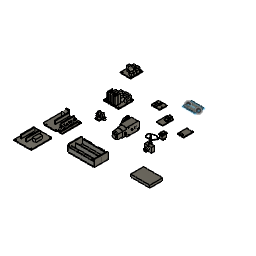
RoboCar2Lib (Autodesk Fusion 360 design; units mm, degrees)
Autodesk Fusion 360 part; units mm, degrees
(part 1 of 2)
sketch "Sketch1" plane through (0, 0, 0) normal (0, 1, 0) x (1, 0, 0)
  line L0 (25, -36.5) -> (33.5, -36.5)
  line L1 (33.5, -36.5) -> (33.5, -13.5)
  line L2 (33.5, -13.5) -> (25, -13.5)
  line L3 (25.0032, -15) -> (25, -15)
  line L4 (32.5, -31.6144) -> (32.5, -18.3856)
  line L5 (25, -36.5) -> (14.5, -36.5)
  line L6 (14.5, -36.5) -> (14.5, -13.5)
  line L7 (14.5, -13.5) -> (25, -13.5)
  line L8 (25, -36.5) -> (16.5, -36.5)
  line L9 (16.5, -32.746) -> (16.5, -17.254)
  line L10 (16.5, -13.5) -> (25, -13.5)
  arc A0 (32.5, -18.3856) -> (17.5, -18.3856) centre (25, -25) ccw
  arc A1 (17.5, -31.6144) -> (32.5, -31.6144) centre (25, -25) ccw
  arc A2 (33.5, -17.254) -> (16.5, -17.254) centre (25, -25) ccw
  arc A3 (16.5, -32.746) -> (33.5, -32.746) centre (25, -25) ccw
  line L11 (17.5, -31.6144) -> (17.5, -18.3856)
  circle A4 centre (25, -25) radius 5
  dimension "d1" = 20
  dimension "d2" = 23
  dimension "d3" = 8.5
  dimension "d4" = 23
  dimension "d7" = 10.5
  dimension "d8" = 23
  dimension "d16" = 10
  constraint concentric A0 A2
  constraint horizontal L0
  constraint vertical L1
  constraint horizontal L2
  constraint coincident L0.start A2
  constraint horizontal L3
  constraint coincident L1 A3.end
  constraint coincident L1 A2.start
  constraint coincident L3.start A0
  constraint horizontal L5
  constraint vertical L6
  constraint horizontal L7
  constraint horizontal L8
  constraint vertical L9
  constraint horizontal L10
  constraint concentric A0 A1
  constraint concentric A2 A3
  constraint concentric A3 A4
  measures "d1" diameter of A0
  measures "d2" diameter of A2
  measures "d3" distance of L0.start L0.end
  measures "d4" distance of L0.start L2.end
  measures "d7" distance of L0.start L5.end
  measures "d8" distance of L0.start L2.end
  measures "d16" diameter of A4
extrude "Extrude1" add sketch "Sketch1" against normal blind 25 contours L3 L4 A0 A1 L11 | A4 makes body 1
extrude "Extrude2" add sketch "Sketch1" against normal blind 11 contours L1 L9 A2 A3 bodies 1
extrude "Extrude3" add sketch "Sketch1" along normal blind 37 contours L0 L1 A3 | L5 L6 L7 L8 L9 L10 A2 A3 | L1 L9 A2 A3 | L1 L2 A2 | L3 L4 A0 A1 L11 | A4 bodies 1
extrude "Extrude4" add sketch "Sketch1" against normal blind 28 contours A4 bodies 1
fillet "Fillet1" radius 4 1 edges at (24, 37, 36.5) on bodies 1
fillet "Fillet2" radius 4 1 edges at (24, 37, 13.5) on bodies 1
sketch "Sketch2" plane through (33.5, 0, 0) normal (1, 0, 0) x (0, 1, 0)
  arc A0 (33, 13.5) -> (37, 17.5) centre (33, 17.5) ccw
  line L0 (37, 17.5) -> (37, 32.5)
  arc A1 (37, 32.5) -> (33, 36.5) centre (33, 32.5) ccw
  line L1 (33, 36.5) -> (0, 36.5)
  line L2 (0, 36.5) -> (0, 32.746)
  line L3 (0, 32.746) -> (-11, 32.746)
  line L4 (-11, 32.746) -> (-11, 17.254)
  line L5 (-11, 17.254) -> (0, 17.254)
  line L6 (0, 17.254) -> (0, 13.5)
  line L7 (0, 13.5) -> (33, 13.5)
  line L8 (0, 36.5) -> (0, 13.5)
  circle A2 centre (14.5, 25) radius 2
  line L9 (0, 25) -> (25.5, 25)
  circle A3 centre (25.5, 25) radius 2.75
  line L10 (0, 25) -> (-11, 25)
  line L11 (-6.5, 27.5) -> (-3.5, 27.5)
  line L12 (-3.5, 27.5) -> (-3.5, 22.5)
  line L13 (-3.5, 22.5) -> (-6.5, 22.5)
  line L14 (-6.5, 22.5) -> (-6.5, 27.5)
  circle A4 centre (5.5, 34) radius 1.5
  circle A5 centre (5.5, 16) radius 1.5
  dimension "d23" = 4
  dimension "d24" = 25.5
  dimension "d25" = 5.5
  dimension "d32" = 4.5
  dimension "d33" = 3
  dimension "d34" = 2.5
  dimension "d35" = 2.5
  dimension "d44" = 3
  dimension "d45" = 5.5
  dimension "d46" = 2.5
  dimension "d47" = 3
  dimension "d48" = 5.5
  dimension "d49" = 2.5
  constraint midpoint L8 L9.start
  constraint perpendicular L8 L9
  constraint coincident L9.end A3.centre
  constraint midpoint L4 L10.end
  constraint horizontal L11
  constraint vertical L12
  constraint horizontal L13
  constraint vertical L14
  measures "d23" diameter of A2
  measures "d24" distance of L9.start L9.end
  measures "d25" diameter of A3
  measures "d32" distance of L4 L14
  measures "d33" distance of L12 L14
  measures "d34" distance of L10 L11
  measures "d35" distance of L10 L13
  measures "d44" diameter of A4
  measures "d45" distance of L8 A4.centre
  measures "d46" distance of L1 A4.centre
  measures "d47" diameter of A5
  measures "d48" distance of L8 A5.centre
  measures "d49" distance of L7 A5.centre
extrude "Extrude5" add sketch "Sketch2" along normal blind 2 contours A2 L9 | A2 L9 bodies 1
extrude "Extrude6" add sketch "Sketch2" along normal blind 8 contours A3 bodies 1
extrude "Extrude7" add sketch "Sketch2" against normal blind 28 contours A3 bodies 1
extrude "Extrude8" add sketch "Sketch2" along normal blind 2.5 contours L10 L12 L13 L14 | L10 L11 L12 L14 bodies 1
extrude "Extrude9" add sketch "Sketch2" against normal blind 19.5 contours L10 L12 L13 L14 | L10 L11 L12 L14 bodies 1
fillet "Fillet3" radius 2 1 edges at (25, -25, 35) on bodies 1
fillet "Fillet4" radius 2 1 edges at (25, -25, 15) on bodies 1
copy_body "Body->Comp1" bodies 1 removing the originals makes body 2 in component "MotorReductor"
extrude "Extrude1'" cut sketch "Sketch2" against normal blind 39 contours A4 | A5 bodies 2 in component "MotorReductor"
sketch "Sketch3" plane through (0, 37, 0) normal (0, 1, 0) x (-1, 0, 0)
  line L0 (-33.5, 17.5) -> (-14.5, 17.5)
  line L1 (-14.5, 17.5) -> (-14.5, 32.5)
  line L2 (-14.5, 32.5) -> (-33.5, 32.5)
  line L3 (-33.5, 32.5) -> (-33.5, 17.5)
  line L4 (-26.5, 27.5) -> (-23.5, 27.5)
  line L5 (-23.5, 27.5) -> (-23.5, 22.5)
  line L6 (-23.5, 22.5) -> (-26.5, 22.5)
  line L7 (-26.5, 22.5) -> (-26.5, 27.5)
  point P0 (-25, 25)
  dimension "d52" = 1.5
  dimension "d53" = 1.5
  dimension "d54" = 2.5
  dimension "d55" = 2.5
  constraint horizontal L4
  constraint vertical L5
  constraint horizontal L6
  constraint vertical L7
  measures "d52" distance of P0 L7
  measures "d53" distance of P0 L5
  measures "d54" distance of P0 L4
  measures "d55" distance of P0 L6
extrude "Extrude2'" add sketch "Sketch3" along normal blind 5 contours L4 L5 L6 L7 bodies 2 in component "MotorReductor"
sketch "Sketch4" plane through (26.5, 0, 0) normal (1, 0, 0) x (0, 1, 0)
  line L0 (37, 27.5) -> (37, 22.5)
  line L1 (37, 22.5) -> (42, 22.5)
  line L2 (42, 22.5) -> (42, 27.5)
  line L3 (42, 27.5) -> (37, 27.5)
  circle A0 centre (39.5, 25) radius 1.5
  dimension "d58" = 3
  measures "d58" diameter of A0
extrude "Extrude3'" cut sketch "Sketch4" against normal blind 9.5 contours A0 bodies 2 in component "MotorReductor"
sketch "Sketch5" plane through (5.5, 0, 0) normal (-1, 0, 0) x (0, -1, 0)
  circle A0 centre (-25.5, 25) radius 2.75
  circle A1 centre (-25.5, 25) radius 13
  line L0 (-26, 36) -> (-25, 36)
  line L1 (-25, 36) -> (-25, 32)
  line L2 (-25, 32) -> (-26, 32)
  line L3 (-26, 32) -> (-26, 36)
  line L4 (-28.1386, 31.5029) -> (-29.3747, 35.3071)
  line L5 (-28.4237, 35.6161) -> (-27.1876, 31.8119)
  line L6 (-29.3747, 35.3071) -> (-28.4237, 35.6161)
  line L7 (-27.1876, 31.8119) -> (-28.1386, 31.5029)
  line L8 (-30.019, 30.3692) -> (-32.3701, 33.6053)
  line L9 (-31.5611, 34.1931) -> (-29.21, 30.957)
  line L10 (-32.3701, 33.6053) -> (-31.5611, 34.1931)
  line L11 (-29.21, 30.957) -> (-30.019, 30.3692)
  line L12 (-31.457, 28.71) -> (-34.6931, 31.0611)
  line L13 (-34.1053, 31.8701) -> (-30.8692, 29.519)
  line L14 (-34.6931, 31.0611) -> (-34.1053, 31.8701)
  line L15 (-30.8692, 29.519) -> (-31.457, 28.71)
  line L16 (-32.3119, 26.6876) -> (-36.1161, 27.9237)
  line L17 (-35.8071, 28.8747) -> (-32.0029, 27.6386)
  line L18 (-36.1161, 27.9237) -> (-35.8071, 28.8747)
  line L19 (-32.0029, 27.6386) -> (-32.3119, 26.6876)
  line L20 (-32.5, 24.5) -> (-36.5, 24.5)
  line L21 (-36.5, 25.5) -> (-32.5, 25.5)
  line L22 (-36.5, 24.5) -> (-36.5, 25.5)
  line L23 (-32.5, 25.5) -> (-32.5, 24.5)
  line L24 (-32.0029, 22.3614) -> (-35.8071, 21.1253)
  line L25 (-36.1161, 22.0763) -> (-32.3119, 23.3124)
  line L26 (-35.8071, 21.1253) -> (-36.1161, 22.0763)
  line L27 (-32.3119, 23.3124) -> (-32.0029, 22.3614)
  line L28 (-30.8692, 20.481) -> (-34.1053, 18.1299)
  line L29 (-34.6931, 18.9389) -> (-31.457, 21.29)
  line L30 (-34.1053, 18.1299) -> (-34.6931, 18.9389)
  line L31 (-31.457, 21.29) -> (-30.8692, 20.481)
  line L32 (-29.21, 19.043) -> (-31.5611, 15.8069)
  line L33 (-32.3701, 16.3947) -> (-30.019, 19.6308)
  line L34 (-31.5611, 15.8069) -> (-32.3701, 16.3947)
  line L35 (-30.019, 19.6308) -> (-29.21, 19.043)
  line L36 (-27.1876, 18.1881) -> (-28.4237, 14.3839)
  line L37 (-29.3747, 14.6929) -> (-28.1386, 18.4971)
  line L38 (-28.4237, 14.3839) -> (-29.3747, 14.6929)
  line L39 (-28.1386, 18.4971) -> (-27.1876, 18.1881)
  line L40 (-25, 18) -> (-25, 14)
  line L41 (-26, 14) -> (-26, 18)
  line L42 (-25, 14) -> (-26, 14)
  line L43 (-26, 18) -> (-25, 18)
  line L44 (-22.8614, 18.4971) -> (-21.6253, 14.6929)
  line L45 (-22.5763, 14.3839) -> (-23.8124, 18.1881)
  line L46 (-21.6253, 14.6929) -> (-22.5763, 14.3839)
  line L47 (-23.8124, 18.1881) -> (-22.8614, 18.4971)
  line L48 (-20.981, 19.6308) -> (-18.6299, 16.3947)
  line L49 (-19.4389, 15.8069) -> (-21.79, 19.043)
  line L50 (-18.6299, 16.3947) -> (-19.4389, 15.8069)
  line L51 (-21.79, 19.043) -> (-20.981, 19.6308)
  line L52 (-19.543, 21.29) -> (-16.3069, 18.9389)
  line L53 (-16.8947, 18.1299) -> (-20.1308, 20.481)
  line L54 (-16.3069, 18.9389) -> (-16.8947, 18.1299)
  line L55 (-20.1308, 20.481) -> (-19.543, 21.29)
  line L56 (-18.6881, 23.3124) -> (-14.8839, 22.0763)
  line L57 (-15.1929, 21.1253) -> (-18.9971, 22.3614)
  line L58 (-14.8839, 22.0763) -> (-15.1929, 21.1253)
  line L59 (-18.9971, 22.3614) -> (-18.6881, 23.3124)
  line L60 (-18.5, 25.5) -> (-14.5, 25.5)
  line L61 (-14.5, 24.5) -> (-18.5, 24.5)
  line L62 (-14.5, 25.5) -> (-14.5, 24.5)
  line L63 (-18.5, 24.5) -> (-18.5, 25.5)
  line L64 (-18.9971, 27.6386) -> (-15.1929, 28.8747)
  line L65 (-14.8839, 27.9237) -> (-18.6881, 26.6876)
  line L66 (-15.1929, 28.8747) -> (-14.8839, 27.9237)
  line L67 (-18.6881, 26.6876) -> (-18.9971, 27.6386)
  line L68 (-20.1308, 29.519) -> (-16.8947, 31.8701)
  line L69 (-16.3069, 31.0611) -> (-19.543, 28.71)
  line L70 (-16.8947, 31.8701) -> (-16.3069, 31.0611)
  line L71 (-19.543, 28.71) -> (-20.1308, 29.519)
  line L72 (-21.79, 30.957) -> (-19.4389, 34.1931)
  line L73 (-18.6299, 33.6053) -> (-20.981, 30.3692)
  line L74 (-19.4389, 34.1931) -> (-18.6299, 33.6053)
  line L75 (-20.981, 30.3692) -> (-21.79, 30.957)
  line L76 (-23.8124, 31.8119) -> (-22.5763, 35.6161)
  line L77 (-21.6253, 35.3071) -> (-22.8614, 31.5029)
  line L78 (-22.5763, 35.6161) -> (-21.6253, 35.3071)
  line L79 (-22.8614, 31.5029) -> (-23.8124, 31.8119)
  dimension "d61" = 26
  dimension "d65" = 360
  constraint concentric A0 A1
  constraint horizontal L0
  constraint vertical L1
  constraint horizontal L2
  constraint vertical L3
  measures "d61" diameter of A1
extrude "Extrude4'" add sketch "Sketch5" against normal blind 3 contours A1 | L0 L1 L2 L3 | L4 L5 L6 L7 | L8 L9 L10 L11 | L12 L13 L14 L15 | L16 L17 L18 L19 | L20 L21 L22 L23 | L24 L25 L26 L27 | L28 L29 L30 L31 | L32 L33 L34 L35 | L36 L37 L38 L39 | L40 L41 L42 L43 | L44 L45 L46 L47 | L48 L49 L50 L51 | L52 L53 L54 L55 | L56 L57 L58 L59 | L60 L61 L62 L63 | L64 L65 L66 L67 | L68 L69 L70 L71 | L72 L73 L74 L75 | L76 L77 L78 L79 bodies 2 in component "MotorReductor"
delete_face "DeleteFace1" 1 faces at (8.5, 15.9753, 24.2175) on bodies 2 in component "MotorReductor"
extrude "Extrude5'" add sketch "Sketch5" against normal blind 3 bodies 2 in component "MotorReductor"
sketch "Sketch6" plane through (0, 0, 0) normal (0, 0, 1) x (1, 0, 0)
  circle A0 centre (-75, 25) radius 1.5
  line L0 (-65, 40) -> (-65, 9)
  line L1 (-75, 21.75) -> (-71, 21.75)
  line L2 (-65, 21.75) -> (-65, 28.25)
  line L3 (-65, 28.25) -> (-75, 28.25)
  line L4 (-65, 21.75) -> (-71, 21.75)
  line L5 (-71, 21.75) -> (-71, 13.75)
  line L6 (-71, 13.75) -> (-65, 13.75)
  line L7 (-65, 13.75) -> (-65, 21.75)
  line L8 (-68, 28.25) -> (-68, 21.75)
  line L9 (-72, 28.25) -> (-72, 21.75)
  arc A1 (-75, 28.25) -> (-75, 21.75) centre (-75, 25) ccw
  circle A2 centre (-69.4791, 26.484) radius 0.8565
  circle A3 centre (-69.4791, 23.583) radius 0.8405
  line L10 (-68.6088, 20.0696) -> (-70.0915, 20.0696)
  line L11 (-70.0915, 20.0696) -> (-70.0915, 17.5876)
  line L12 (-70.0915, 17.5876) -> (-68.6088, 17.5876)
  line L13 (-68.6088, 17.5876) -> (-68.6088, 20.0696)
  line L14 (-66, 16) -> (-70.0593, 16)
  line L15 (-70.0593, 16) -> (-70.0593, 14.6866)
  line L16 (-70.0593, 14.6866) -> (-66, 14.6866)
  line L17 (-66, 14.6866) -> (-66, 16)
  dimension "d68" = 3
  dimension "d69" = 10
  dimension "d70" = 6.5
  dimension "d71" = 6.5
  dimension "d72" = 6
  dimension "d73" = 8
  dimension "d74" = 3
  dimension "d75" = 4
  constraint vertical L0
  constraint concentric A0 A1
  constraint horizontal L1
  constraint vertical L2
  constraint horizontal L3
  constraint horizontal L4
  constraint vertical L5
  constraint horizontal L6
  constraint vertical L7
  constraint coincident L3 L8.start
  constraint coincident L4 L8.end
  constraint perpendicular L4 L8
  constraint coincident L3 L9.start
  constraint coincident L1 L9.end
  constraint perpendicular L1 L9
  constraint horizontal L10
  constraint vertical L11
  constraint horizontal L12
  constraint vertical L13
  constraint horizontal L14
  constraint vertical L15
  constraint horizontal L16
  constraint vertical L17
  measures "d68" diameter of A0
  measures "d69" distance of A0.centre L0
  measures "d70" diameter of A1
  measures "d71" distance of L1.start L3.end
  measures "d72" distance of L2.start L1.end
  measures "d73" distance of L2.start L6.end
  measures "d74" distance of L0 L8
  measures "d75" distance of L8 L9
extrude "Extrude10" add sketch "Sketch6" along normal blind 4.5 separate body contours L1 L3 L9 A1 makes body 3
extrude "Extrude11" add sketch "Sketch6" along normal blind 5 separate body contours L0 L2 L3 L4 L8 makes body 4
extrude "Extrude12" add sketch "Sketch6" along normal blind 13 contours L1 L3 L4 L8 L9 | A2 | A3 bodies 3 4
extrude "Extrude13" add sketch "Sketch6" along normal blind 1.6 contours L0 L4 L5 L6 L7 | L10 L11 L12 L13 | L14 L15 L16 L17 bodies 3
extrude "Extrude14" add sketch "Sketch6" against normal blind 1.3 contours A2 | A3 | L10 L11 L12 L13 | L14 L15 L16 L17 bodies 3
mirror "Mirror1" about plane through (-65, 21.75, 0) normal (1, 0, 0) of bodies 3 merged
copy_body "Body->Comp2" bodies 3 removing the originals makes body 5 in component "Encoder"
sketch "Sketch7" plane through (0, 0, 0) normal (0, 0, 1) x (1, 0, 0)
  line L0 (-26.5653, -67.5474) -> (49.4347, -67.5474)
  line L1 (49.4347, -67.5474) -> (49.4347, -108.5474)
  line L2 (49.4347, -108.5474) -> (-26.5653, -108.5474)
  line L3 (-26.5653, -108.5474) -> (-26.5653, -67.5474)
  line L4 (47.4347, -67.5474) -> (47.4347, -108.5474)
  line L5 (-24.5653, -67.5474) -> (-24.5653, -108.5474)
  dimension "d88" = 76
  dimension "d89" = 41
  dimension "d90" = 2
  dimension "d91" = 2
  constraint horizontal L0
  constraint vertical L1
  constraint horizontal L2
  constraint vertical L3
  constraint perpendicular L2 L4
  constraint coincident L0 L4.start
  constraint coincident L2 L4.end
  constraint vertical L5
  constraint coincident L0 L5.start
  constraint coincident L2 L5.end
  measures "d88" distance of L0.start L0.end
  measures "d89" distance of L0.start L2.end
  measures "d90" distance of L1 L4
  measures "d91" distance of L3 L5
extrude "Extrude15" add sketch "Sketch7" along normal blind 20 separate body contours L0 L2 L3 L5 | L0 L1 L2 L4 makes body 6 at (-24.5653, -81.2141, 6.6667) makes body 7 at (49.4347, -81.2141, 6.6667)
extrude "Extrude16" add sketch "Sketch7" along normal blind 2 contours L0 L2 L4 L5 bodies 6 7
fillet "Fillet5" radius 4 4 edges at (48.4347, -108.5474, 20) (-25.5653, -108.5474, 20) (48.4347, -67.5474, 20) (-25.5653, -67.5474, 20) on bodies 6
sketch "Sketch8" plane through (-26.5653, 0, 0) normal (-1, 0, 0) x (0, -1, 0)
  arc A0 (71.5474, 20) -> (67.5474, 16) centre (71.5474, 16) ccw
  line L0 (67.5474, 16) -> (67.5474, 0)
  line L1 (67.5474, 0) -> (108.5474, 0)
  line L2 (108.5474, 0) -> (108.5474, 16)
  arc A1 (108.5474, 16) -> (104.5474, 20) centre (104.5474, 16) ccw
  line L3 (104.5474, 20) -> (71.5474, 20)
  line L4 (108.5474, 0) -> (107.0474, 0)
  line L5 (107.0474, 0) -> (107.0474, 14)
  line L6 (108.5474, 14) -> (108.5474, 0)
  line L7 (67.5474, 0) -> (69.0474, 0)
  line L8 (69.0474, 0) -> (69.0474, 14)
  line L9 (67.5474, 14) -> (67.5474, 0)
  arc A2 (70.1082, 18.3088) -> (67.5474, 14) centre (72.4529, 14) ccw
  arc A3 (70.7763, 16.9642) -> (69.0474, 14) centre (72.4529, 14) ccw
  line L10 (70.6663, 18.1167) -> (70.9463, 17.4716)
  arc A4 (70.6663, 18.1167) -> (70.1082, 18.3088) centre (70.2994, 17.9575) ccw
  arc A5 (70.7763, 16.9642) -> (70.9463, 17.4716) centre (70.5794, 17.3123) ccw
  line L11 (88.0474, 20) -> (88.0474, 0)
  arc A6 (108.5474, 14) -> (105.9866, 18.3088) centre (103.6419, 14) ccw
  arc A7 (107.0474, 14) -> (105.3185, 16.9642) centre (103.6419, 14) ccw
  arc A8 (105.9866, 18.3088) -> (105.4285, 18.1167) centre (105.7955, 17.9575) ccw
  line L12 (105.4285, 18.1167) -> (105.1485, 17.4716)
  arc A9 (105.1485, 17.4716) -> (105.3185, 16.9642) centre (105.5155, 17.3123) ccw
  line L13 (87.3474, 14) -> (88.7474, 14)
  line L14 (108.5474, 0) -> (67.5474, 0)
  line L15 (88.7474, 14) -> (88.7474, 0)
  line L16 (87.3474, 14) -> (87.3474, 0)
  dimension "d98" = 1.5
  dimension "d99" = 14
  dimension "d100" = 1.5
  dimension "d102" = 0.4
  dimension "d103" = 20.5
  dimension "d106" = 14
  constraint horizontal L4
  constraint vertical L5
  constraint vertical L6
  constraint coincident L1.end L2.start
  constraint horizontal L7
  constraint vertical L8
  constraint vertical L9
  constraint coincident L0.end L1.start
  constraint tangent L9 A2
  constraint concentric A2 A3
  constraint tangent A2 A4
  constraint tangent L10 A4
  constraint tangent A3 A5
  constraint tangent L10 A5
  constraint equal A4 A5
  constraint perpendicular L1 L11
  constraint symmetric L9.start L11 L6.start
  constraint symmetric A2 L11 A6
  constraint symmetric L8.end L11 L5.end
  constraint symmetric A3 L11 A7
  constraint symmetric L10.start L11 A8.end
  constraint symmetric A2.start L11 A6.end
  constraint symmetric A4 L11 A8
  constraint symmetric L10.end L11 L12.end
  constraint symmetric A3.start L11 A7.end
  constraint symmetric A5 L11 A9
  constraint coincident L1 L11.end
  constraint coincident L3 L11.start
  constraint coincident L1 L15.end
  constraint coincident L1 L16.end
  measures "d98" distance of L1.end L4.end
  measures "d99" distance of L1.end L6.start
  measures "d100" distance of L0.end L7.end
  measures "d102" radius of A4
  measures "d103" distance of L9 L11
  measures "d106" distance of L13 L14
extrude "Extrude17" add sketch "Sketch8" against normal blind 74 contours L0 L1 L7 L8 L9 A2 A3 L10 A4 A5 L14 | L1 L11 L13 L14 L15 | L1 L11 L13 L14 L16 | L1 L2 L4 L5 L6 A6 A7 A8 L12 A9 L14 bodies 6
sketch "Sketch9" plane through (0, -108.5474, 0) normal (0, -1, 0) x (1, 0, 0)
  line L0 (-24.5653, 14) -> (-24.5653, 16)
  line L1 (-24.5653, 16) -> (-26.5653, 16)
  line L2 (-26.5653, 16) -> (-26.5653, 0)
  line L3 (-26.5653, 0) -> (49.4347, 0)
  line L4 (49.4347, 0) -> (49.4347, 16)
  line L5 (49.4347, 16) -> (47.4347, 16)
  line L6 (47.4347, 16) -> (47.4347, 14)
  line L7 (47.4347, 14) -> (-24.5653, 14)
  line L8 (4.284, 14) -> (18.5854, 14)
  line L9 (49.4347, 0) -> (-26.5653, 0)
  line L10 (3.4347, 14.2636) -> (3.4347, 14)
  line L11 (19.4347, 14.2636) -> (19.4347, 14)
  line L12 (0.4347, 19) -> (2.9978, 14.7283)
  line L13 (22.4347, 19) -> (19.8717, 14.7283)
  arc A0 (2.9978, 14.7283) -> (4.284, 14) centre (4.284, 15.5) ccw
  arc A1 (18.5854, 14) -> (19.8717, 14.7283) centre (18.5854, 15.5) ccw
  line L14 (0.4347, 19) -> (22.4347, 19)
  line L15 (-26.5653, 16) -> (-26.5653, 20)
  line L16 (-18.5653, 17) -> (-18.5653, 20)
  line L17 (-18.5653, 20) -> (-24.5653, 20)
  line L18 (-24.5653, 20) -> (-24.5653, 17)
  arc A2 (-24.5653, 17) -> (-18.5653, 17) centre (-21.5653, 17) ccw
  line L19 (47.4347, 17) -> (47.4347, 20)
  line L20 (47.4347, 20) -> (41.4347, 20)
  line L21 (41.4347, 20) -> (41.4347, 17)
  arc A3 (41.4347, 17) -> (47.4347, 17) centre (44.4347, 17) ccw
  dimension "d109" = 14
  dimension "d115" = 1.5
  dimension "d116" = 6
  dimension "d117" = 5
  dimension "d118" = 6
  dimension "d119" = 6
  dimension "d120" = 5
  dimension "d121" = 6
  dimension "d122" = 3
  constraint horizontal L8
  constraint vertical L10
  constraint vertical L11
  constraint tangent L12 A0
  constraint tangent L8 A0
  constraint tangent L13 A1
  constraint tangent L8 A1
  constraint equal A0 A1
  constraint coincident A0 L10.start
  constraint coincident L7 L10.end
  constraint coincident L7 L11.end
  constraint coincident A1 L11.start
  constraint vertical L16
  constraint horizontal L17
  constraint vertical L18
  constraint vertical L19
  constraint horizontal L20
  constraint vertical L21
  measures "d109" distance of L8 L9
  measures "d115" radius of A0
  measures "d116" diameter of A2
  measures "d117" distance of A2.centre L15
  measures "d118" distance of L18.end L16.start
  measures "d119" diameter of A3
  measures "d120" distance of L4 A3.centre
  measures "d121" distance of L21.end L19.start
  measures "d122" distance of L21.end L20.end
extrude "Extrude18" cut sketch "Sketch9" against normal blind 45 contours L16 L17 L18 A2 | L19 L20 L21 A3 | L7 L8 L12 L13 A0 A1 L14 bodies 6
copy_body "Body->Comp3" bodies 6 removing the originals makes body 8 in component "BattaryHolder"
sketch "Sketch10" plane through (0, 0, 0) normal (0, 0, 1) x (1, 0, 0)
  line L0 (-134.5632, -15) -> (-80.9632, -15)
  line L1 (-80.9632, -15) -> (-80.9632, -70)
  line L2 (-97.4, -73) -> (-130, -73)
  line L3 (-134.5632, -70) -> (-134.5632, -15)
  line L4 (-130, -73) -> (-133, -70)
  line L5 (-94.4, -70) -> (-97.4, -73)
  line L6 (-94.4, -70) -> (-98.6426, -70) construction
  line L7 (-134.5632, -70) -> (-133, -70)
  line L8 (-94.4, -70) -> (-80.9632, -70)
  circle A0 centre (-131.5632, -19.5) radius 1.5
  circle A1 centre (-83.9632, -19.5) radius 1.5
  circle A2 centre (-126.5632, -70.5) radius 1.5
  circle A3 centre (-98.9632, -70.5) radius 1.5
  line L9 (-127.5632, -12) -> (-118.5632, -12)
  line L10 (-118.5632, -12) -> (-118.5632, -26)
  line L11 (-118.5632, -26) -> (-127.5632, -26)
  line L12 (-127.5632, -26) -> (-127.5632, -12)
  line L13 (-116.0632, -17.5) -> (-113.5632, -17.5)
  line L14 (-113.5632, -17.5) -> (-113.5632, -56.5)
  line L15 (-113.5632, -56.5) -> (-116.0632, -56.5)
  line L16 (-116.0632, -56.5) -> (-116.0632, -17.5)
  line L17 (-100.5632, -17.5) -> (-98.0632, -17.5)
  line L18 (-98.0632, -17.5) -> (-98.0632, -56.5)
  line L19 (-98.0632, -56.5) -> (-100.5632, -56.5)
  line L20 (-100.5632, -56.5) -> (-100.5632, -17.5)
  line L21 (-93.9632, -20) -> (-86.4632, -20)
  line L22 (-86.4632, -20) -> (-86.4632, -30)
  line L23 (-86.4632, -30) -> (-93.9632, -30)
  line L24 (-93.9632, -30) -> (-93.9632, -20)
  circle A4 centre (-92.7132, -21.25) radius 0.5
  circle A5 centre (-90.2132, -21.25) radius 0.5
  circle A6 centre (-87.7132, -21.25) radius 0.5
  circle A7 centre (-92.7132, -23.75) radius 0.5
  circle A8 centre (-90.2132, -23.75) radius 0.5
  circle A9 centre (-87.7132, -23.75) radius 0.5
  circle A10 centre (-92.7132, -26.25) radius 0.5
  circle A11 centre (-90.2132, -26.25) radius 0.5
  circle A12 centre (-87.7132, -26.25) radius 0.5
  circle A13 centre (-92.7132, -28.75) radius 0.5
  circle A14 centre (-90.2132, -28.75) radius 0.5
  circle A15 centre (-87.7132, -28.75) radius 0.5
  dimension "d125" = 53.6
  dimension "d126" = 58
  dimension "d127" = 3
  dimension "d129" = 45
  dimension "d130" = 3
  dimension "d131" = 3
  dimension "d132" = 3
  dimension "d133" = 3
  dimension "d134" = 3
  dimension "d135" = 3
  dimension "d136" = 4.5
  dimension "d137" = 4.5
  dimension "d138" = 2.5
  dimension "d139" = 2.5
  dimension "d140" = 8
  dimension "d141" = 18
  dimension "d142" = 7
  dimension "d143" = 9
  dimension "d144" = 3
  dimension "d145" = 14
  dimension "d146" = 18.5
  dimension "d147" = 2.5
  dimension "d148" = 2.5
  dimension "d149" = 2.5
  dimension "d150" = 39
  dimension "d151" = 39
  dimension "d152" = 13
  dimension "d153" = 2.5
  dimension "d154" = 5
  dimension "d155" = 5.5
  dimension "d156" = 7.5
  dimension "d157" = 10
  dimension "d158" = 1
  dimension "d159" = 1.25
  dimension "d160" = 1.25
  dimension "d163" = 5
  dimension "d164" = -7.5
  constraint horizontal L0
  constraint vertical L1
  constraint horizontal L2
  constraint vertical L3
  constraint perpendicular L1 L7
  constraint coincident L5.start L7
  constraint horizontal L6
  constraint collinear L7 L8
  constraint horizontal L9
  constraint vertical L10
  constraint horizontal L11
  constraint vertical L12
  constraint horizontal L13
  constraint vertical L14
  constraint horizontal L15
  constraint vertical L16
  constraint horizontal L17
  constraint vertical L18
  constraint horizontal L19
  constraint vertical L20
  constraint horizontal L21
  constraint vertical L22
  constraint horizontal L23
  constraint vertical L24
  measures "d125" distance of L0.start L0.end
  measures "d126" distance of L0 L2
  measures "d127" distance of L2 L7
  measures "d129" angle of L5 L6
  measures "d130" diameter of A0
  measures "d131" diameter of A1
  measures "d132" diameter of A2
  measures "d133" diameter of A3
  measures "d134" distance of L3 A0.centre
  measures "d135" distance of L1 A1.centre
  measures "d136" distance of L0 A0.centre
  measures "d137" distance of L0 A1.centre
  measures "d138" distance of L2 A2.centre
  measures "d139" distance of L2 A3.centre
  measures "d140" distance of L3 A2.centre
  measures "d141" distance of L1 A3.centre
  measures "d142" distance of L3 L12
  measures "d143" distance of L10 L12
  measures "d144" distance of L0 L9
  measures "d145" distance of L9 L11
  measures "d146" distance of L3 L16
  measures "d147" distance of L14 L16
  measures "d148" distance of L0 L13
  measures "d149" distance of L0 L17
  measures "d150" distance of L13 L15
  measures "d151" distance of L17 L19
  measures "d152" distance of L14 L20
  measures "d153" distance of L18 L20
  measures "d154" distance of L0 L21
  measures "d155" distance of L1 L22
  measures "d156" distance of L22 L24
  measures "d157" distance of L21 L23
  measures "d158" diameter of A4
  measures "d159" distance of L21 A4.centre
  measures "d160" distance of L24 A4.centre
extrude "Extrude19" add sketch "Sketch10" against normal blind 1.7 separate body contours L0 L1 L2 L3 L4 L5 L7 L8 L10 L11 L12 | L0 L10 L11 L12 | A0 | A1 | A2 | A3 | L13 L14 L15 L16 | L17 L18 L19 L20 | L21 L22 L23 L24 | A4 | A5 | A6 | A7 | A8 | A9 | A10 | A11 | A12 | A13 | A14 | A15 makes body 9
extrude "Extrude20" add sketch "Sketch10" along normal blind 11 contours L0 L9 L10 L12 | L0 L10 L11 L12 bodies 9
extrude "Extrude21" add sketch "Sketch10" along normal blind 8.5 contours L13 L14 L15 L16 | L17 L18 L19 L20 bodies 9
extrude "Extrude22" add sketch "Sketch10" along normal blind 8 contours A4 | A5 | A6 | A7 | A8 | A9 | A10 | A11 | A12 | A13 | A14 | A15 bodies 9
extrude "Extrude23" add sketch "Sketch10" along normal blind 2.5 contours L21 L22 L23 L24 bodies 9
pattern_linear "R-Pattern1" count 4 spacing 12.6667 along (0, -1, 0) of 29 faces at (-87.3641, -20.892, 4.3333) (-90.0484, -23.7748, 8) (-92.5484, -26.2748, 8) (-92.5484, -23.7748, 8) (-92.3641, -28.392, 4.3333) (-87.5484, -21.2748, 8) (-87.3641, -28.392, 4.3333) (-89.8641, -23.392, 4.3333) (-92.3641, -23.392, 4.3333) (-87.5484, -26.2748, 8) (-89.8641, -28.392, 4.3333) (-92.5484, -28.7748, 8) (-92.5484, -21.2748, 8) (-87.5484, -28.7748, 8) (-87.5484, -23.7748, 8) (-92.3641, -25.892, 4.3333) (-92.3641, -20.892, 4.3333) (-87.3641, -23.392, 4.3333) (-90.0484, -21.2748, 8) (-90.0484, -28.7748, 8) (-89.8641, -25.892, 4.3333) (-90.0484, -26.2748, 8) (-91.7577, -27.1967, 2.5) (-89.8641, -20.892, 4.3333) (-87.3641, -25.892, 4.3333) (-91.4632, -20, 0.8333) (-86.4632, -23.3333, 0.8333) (-88.9632, -30, 0.8333) (-93.9632, -26.6666, 0.8333) on bodies 9
sketch "Sketch11" plane through (0, -26, 0) normal (0, -1, 0) x (1, 0, 0)
  line L0 (-127.5632, 0) -> (-118.5632, 0)
  line L1 (-118.5632, 0) -> (-118.5632, 11)
  line L2 (-118.5632, 11) -> (-127.5632, 11)
  line L3 (-127.5632, 11) -> (-127.5632, 0)
  line L4 (-127.5632, 11) -> (-118.5632, 11)
  line L5 (-118.5632, 11) -> (-118.5632, 6.5)
  line L6 (-127.5632, 6.5) -> (-127.5632, 11)
  arc A0 (-118.5632, 6.5) -> (-127.5632, 6.5) centre (-123.0632, 6.5) ccw
  line L7 (-118.5632, 5.5) -> (-118.6757, 5.5)
  dimension "d179" = 9
  dimension "d180" = 4.5
  constraint horizontal L4
  constraint vertical L5
  constraint horizontal L7
  constraint vertical L6
  constraint midpoint L1 L7.start
  constraint coincident L2.end L3.start
  constraint coincident L3 L6.start
  constraint coincident L1 L5.end
  measures "d179" diameter of A0
  measures "d180" distance of L2 A0.centre
extrude "Extrude24" cut sketch "Sketch11" against normal blind 11 contours L2 L3 L4 L6 A0 | L1 L2 L4 L5 A0 bodies 9
copy_body "Body->Comp4" bodies 9 removing the originals makes body 10 in component "MaketNano"
ref_plane "WorkPlane1" through (-114.8132, -37, 30.5) normal (0, 0, 1) x (1, 0, 0)
sketch "Sketch12" plane through (0, 0, 30.5) normal (0, 0, 1) x (1, 0, 0)
  line L0 (-116.0632, -56.5) -> (-113.5632, -56.5)
  line L1 (-113.5632, -56.5) -> (-113.5632, -17.5)
  line L2 (-113.5632, -17.5) -> (-116.0632, -17.5)
  line L3 (-116.0632, -17.5) -> (-116.0632, -56.5)
  line L4 (-100.5632, -56.5) -> (-98.0632, -56.5)
  line L5 (-98.0632, -56.5) -> (-98.0632, -17.5)
  line L6 (-98.0632, -17.5) -> (-100.5632, -17.5)
  line L7 (-100.5632, -17.5) -> (-100.5632, -56.5)
  line L8 (-98.0632, -17.5) -> (-116.0632, -17.5)
  line L9 (-116.0632, -17.5) -> (-116.0632, -56.5)
  line L10 (-116.0632, -56.5) -> (-98.0632, -56.5)
  line L11 (-98.0632, -56.5) -> (-98.0632, -17.5)
  constraint horizontal L8
  constraint vertical L9
  constraint horizontal L10
  constraint vertical L11
  constraint coincident L0.start L3.end
  constraint coincident L5.end L6.start
extrude "Extrude1''" cut sketch "Sketch10" against normal blind 2.5 contours A0 | A1 | A2 | A3 bodies 10 in component "MaketNano"
sketch "Sketch13" plane through (0, 0, 0) normal (0, 0, 1) x (1, 0, 0)
  line L0 (-61.7349, 72.3961) -> (-105.2349, 72.3961)
  line L1 (-105.2349, 72.3961) -> (-105.2349, 115.8961)
  line L2 (-105.2349, 115.8961) -> (-61.7349, 115.8961)
  line L3 (-61.7349, 115.8961) -> (-61.7349, 72.3961)
  circle A0 centre (-65.2349, 75.8961) radius 1.5
  circle A1 centre (-101.7349, 75.8961) radius 1.5
  circle A2 centre (-65.2349, 112.3961) radius 1.5
  circle A3 centre (-101.7349, 112.3961) radius 1.5
  line L4 (-71.7349, 72.3961) -> (-95.2349, 72.3961)
  line L5 (-95.2349, 72.3961) -> (-95.2349, 88.1961)
  line L6 (-71.7349, 88.1961) -> (-71.7349, 72.3961)
  line L7 (-72.4349, 81.1961) -> (-94.5349, 81.1961)
  line L8 (-71.7349, 72.3961) -> (-72.4349, 72.3961)
  line L9 (-71.7349, 80.576) -> (-71.7349, 72.3961)
  line L10 (-95.2349, 72.3961) -> (-94.5349, 72.3961)
  line L11 (-95.2349, 80.576) -> (-95.2349, 72.3961)
  line L12 (-75.9349, 72.3961) -> (-76.6349, 72.3961)
  line L13 (-76.6349, 72.3961) -> (-76.6349, 80.576)
  line L14 (-75.9349, 80.576) -> (-75.9349, 72.3961)
  line L15 (-80.4349, 72.3961) -> (-81.1349, 72.3961)
  line L16 (-81.1349, 72.3961) -> (-81.1349, 80.576)
  line L17 (-80.4349, 80.576) -> (-80.4349, 72.3961)
  line L18 (-85.8349, 72.3961) -> (-86.5349, 72.3961)
  line L19 (-86.5349, 72.3961) -> (-86.5349, 80.576)
  line L20 (-85.8349, 80.576) -> (-85.8349, 72.3961)
  line L21 (-90.3349, 72.3961) -> (-91.0349, 72.3961)
  line L22 (-91.0349, 72.3961) -> (-91.0349, 80.576)
  line L23 (-90.3349, 80.576) -> (-90.3349, 72.3961)
  line L24 (-105.2349, 96.3961) -> (-97.2349, 96.3961)
  line L25 (-97.2349, 96.3961) -> (-97.2349, 106.3961)
  line L26 (-97.2349, 106.3961) -> (-105.2349, 106.3961)
  line L27 (-105.2349, 106.3961) -> (-105.2349, 96.3961)
  line L28 (-94.5349, 72.3961) -> (-94.5349, 80.576)
  line L29 (-94.5349, 81.1961) -> (-94.5349, 88.1961)
  line L30 (-91.0349, 80.576) -> (-94.5349, 80.576)
  line L31 (-86.5349, 80.576) -> (-90.3349, 80.576)
  line L32 (-72.4349, 80.576) -> (-75.9349, 80.576)
  line L33 (-76.6349, 80.576) -> (-80.4349, 80.576)
  line L34 (-81.1349, 80.576) -> (-85.8349, 80.576)
  line L35 (-72.4349, 72.3961) -> (-72.4349, 80.576)
  line L36 (-72.4349, 81.1961) -> (-72.4349, 88.1961)
  line L37 (-95.2349, 88.1961) -> (-94.5349, 88.1961)
  line L38 (-72.4349, 88.1961) -> (-71.7349, 88.1961)
  circle A4 centre (-77, 96) radius 4
  line L39 (-98.9871, 115.8961) -> (-83.9871, 115.8961)
  line L40 (-83.9871, 115.8961) -> (-83.9871, 110.8961)
  line L41 (-83.9871, 110.8961) -> (-98.9871, 110.8961)
  line L42 (-98.9871, 110.8961) -> (-98.9871, 115.8961)
  circle A5 centre (-85.2371, 114.6461) radius 0.5
  circle A6 centre (-87.7371, 114.6461) radius 0.5
  circle A7 centre (-90.2371, 114.6461) radius 0.5
  circle A8 centre (-92.7371, 114.6461) radius 0.5
  circle A9 centre (-95.2371, 114.6461) radius 0.5
  circle A10 centre (-97.7371, 114.6461) radius 0.5
  circle A11 centre (-85.2371, 112.1461) radius 0.5
  circle A12 centre (-97.7371, 112.1461) radius 0.5
  circle A13 centre (-90, 106) radius 4
  dimension "d186" = 43.5
  dimension "d187" = 43.5
  dimension "d188" = 3
  dimension "d189" = 3
  dimension "d190" = 3
  dimension "d191" = 3
  dimension "d192" = 3.5
  dimension "d193" = 3.5
  dimension "d194" = 3.5
  dimension "d195" = 3.5
  dimension "d196" = 3.5
  dimension "d197" = 3.5
  dimension "d198" = 3.5
  dimension "d199" = 3.5
  dimension "d200" = 23.5
  dimension "d201" = 15.8
  dimension "d202" = 10
  dimension "d203" = 7
  dimension "d205" = 0.7
  dimension "d206" = 0.7
  dimension "d207" = 0.7
  dimension "d208" = 0.7
  dimension "d209" = 0.7
  dimension "d210" = 0.7
  dimension "d211" = 3.5
  dimension "d212" = 8
  dimension "d213" = 8
  dimension "d214" = 3.5
  dimension "d215" = 8
  dimension "d216" = 10
  dimension "d217" = 9.5
  dimension "d227" = 8
  dimension "d228" = 15
  dimension "d229" = 5
  dimension "d230" = 1
  dimension "d231" = 1.25
  dimension "d232" = 1.25
  dimension "d235" = -12.5
  dimension "d236" = 0
  dimension "d247" = 8
  constraint horizontal L0
  constraint vertical L1
  constraint horizontal L2
  constraint vertical L3
  constraint horizontal L4
  constraint vertical L5
  constraint horizontal L37
  constraint vertical L6
  constraint coincident L0 L4.start
  constraint perpendicular L5 L7
  constraint horizontal L8
  constraint vertical L35
  constraint vertical L9
  constraint horizontal L10
  constraint vertical L28
  constraint vertical L11
  constraint horizontal L12
  constraint vertical L13
  constraint vertical L14
  constraint coincident L4 L12.start
  constraint horizontal L15
  constraint vertical L16
  constraint vertical L17
  constraint coincident L0 L15.start
  constraint horizontal L18
  constraint vertical L19
  constraint vertical L20
  constraint coincident L4 L18.start
  constraint horizontal L21
  constraint vertical L22
  constraint vertical L23
  constraint coincident L0 L21.start
  constraint horizontal L24
  constraint vertical L25
  constraint horizontal L26
  constraint vertical L27
  constraint coincident L1 L24.start
  constraint coincident L36.end L37
  constraint coincident L7.end L28
  constraint collinear L28 L29
  constraint collinear L30 L32
  constraint collinear L31 L32
  constraint collinear L32 L33
  constraint collinear L33 L34
  constraint coincident L7.start L35
  constraint collinear L35 L36
  constraint collinear L37 L38
  constraint horizontal L39
  constraint vertical L40
  constraint horizontal L41
  constraint vertical L42
  constraint coincident L2 L39.start
  measures "d186" distance of L0.start L0.end
  measures "d187" distance of L0.start L2.end
  measures "d188" diameter of A0
  measures "d189" diameter of A1
  measures "d190" diameter of A2
  measures "d191" diameter of A3
  measures "d192" distance of L3 A0.centre
  measures "d193" distance of L0 A0.centre
  measures "d194" distance of L0 A1.centre
  measures "d195" distance of L1 A1.centre
  measures "d196" distance of L1 A3.centre
  measures "d197" distance of L2 A3.centre
  measures "d198" distance of L2 A2.centre
  measures "d199" distance of L3 A2.centre
  measures "d200" distance of L4.start L4.end
  measures "d201" distance of L4.start L6.start
  measures "d202" distance of L3 L6
  measures "d203" distance of L7 L37
  measures "d205" distance of L4.start L8.end
  measures "d206" distance of L4.end L10.end
  measures "d207" distance of L12.start L12.end
  measures "d208" distance of L15.start L15.end
  measures "d209" distance of L18.start L18.end
  measures "d210" distance of L21.start L21.end
  measures "d211" distance of L14 L35
  measures "d212" distance of L17 L35
  measures "d213" distance of L19 L28
  measures "d214" distance of L22 L28
  measures "d215" distance of L24.start L24.end
  measures "d216" distance of L24.start L26.end
  measures "d217" distance of L2 L26
  measures "d227" diameter of A4
  measures "d228" distance of L39.start L39.end
  measures "d229" distance of L39.start L41.end
  measures "d230" diameter of A5
  measures "d231" distance of L40 A5.centre
  measures "d232" distance of L39 A5.centre
  measures "d247" diameter of A13
extrude "Extrude25" add sketch "Sketch13" against normal blind 1.6 separate body contours L0 L1 L2 L3 L5 L6 L7 L9 L11 L24 L25 L26 L29 L36 L37 L38 L40 L41 L42 | L0 L4 L5 L6 L7 L8 L9 L10 L11 L12 L13 L14 L15 L16 L17 L18 L19 L20 L21 L22 L23 L28 L29 L30 L31 L32 L33 L34 L35 L36 L37 L38 | L0 L4 L14 L32 L35 | L2 L39 L40 L41 L42 | L0 L4 L13 L17 L33 | L1 L24 L25 L26 L27 | L0 L4 L16 L20 L34 | L0 L4 L19 L23 L31 | L0 L4 L22 L28 L30 | A4 | A5 | A6 | A7 | A8 | A9 | A10 | A11 | A12 | A13 makes body 11
extrude "Extrude26" add sketch "Sketch13" along normal blind 25 contours L0 L4 L5 L6 L7 L8 L9 L10 L11 L12 L13 L14 L15 L16 L17 L18 L19 L20 L21 L22 L23 L28 L29 L30 L31 L32 L33 L34 L35 L36 L37 L38 bodies 11
extrude "Extrude27" add sketch "Sketch13" along normal blind 10 separate body contours L1 L24 L25 L26 L27 makes body 12
chamfer "Chamfer1" distance 1.5 distance2 4 2 edges at (-97.2349, 101.3961, 10) (-105.2349, 101.3961, 10) measured on face at (-99.9015, 103.0628, 10) measured on face at (-99.9015, 103.0628, 10) on bodies 12
copy_body "CopyPasteBodies1" bodies 12 makes body 13
move_body "Move1" bodies 13 to x (1, 0, 0) y (0, 1, 0) z (0, 0, 1) at (35.4, 0, 0)
copy_body "CopyPasteBodies2" bodies 13 makes body 14
move_body "Move2" bodies 14 to x (0, 1, 0) y (-1, 0, 0) z (0, 0, 1) at (28.0612, 177.731, 0)
move_face "OffsetFaces1" offset 5 1 faces at (-78.3349, 110.5628, 4) on bodies 14
extrude "Extrude28" add sketch "Sketch13" along normal blind 8 contours A5 | A6 | A7 | A8 | A9 | A10 | A11 | A12 bodies 11
extrude "Extrude29" add sketch "Sketch13" along normal blind 2.5 contours L2 L39 L40 L41 L42 bodies 11
extrude "Extrude30" add sketch "Sketch13" along normal blind 10 contours A4 bodies 11
extrude "Extrude31" add sketch "Sketch13" along normal blind 10 contours A13 bodies 11
combine "Combine1" operation add target body 11 tool bodies 12 13 14
copy_body "Body->Comp5" bodies 11 removing the originals makes body 15 in component "MotorDriver"
sketch "Sketch14" plane through (0, 0, 0) normal (0, 0, 1) x (1, 0, 0)
  line L0 (-25, 150) -> (-0.3, 150)
  line L1 (-0.3, 150) -> (-0.3, 128.9)
  line L2 (-0.3, 128.9) -> (-25, 128.9)
  line L3 (-25, 128.9) -> (-25, 150)
  circle A0 centre (-2.8, 137.4) radius 1.5
  line L4 (-17.5, 137.4) -> (-14, 137.4)
  line L5 (-12.5, 135.9) -> (-12.5, 130.9)
  line L6 (-12.5, 130.9) -> (-19, 130.9)
  line L7 (-19, 130.9) -> (-19, 135.9)
  line L8 (-14, 137.4) -> (-12.5, 135.9)
  line L9 (-17.5, 137.4) -> (-19, 135.9)
  circle A1 centre (-15.7, 134.1) radius 3.2
  line L10 (-15, 148) -> (-11, 148)
  line L11 (-11, 148) -> (-11, 138)
  line L12 (-11, 138) -> (-15, 138)
  line L13 (-15, 138) -> (-15, 148)
  point P0 (-19, 137.4)
  point P1 (-12.5, 137.4)
  dimension "d250" = 24.7
  dimension "d251" = 21.1
  dimension "d252" = 3
  dimension "d253" = 8.5
  dimension "d254" = 2.5
  dimension "d255" = 6.5
  dimension "d256" = 6.5
  dimension "d258" = 2
  dimension "d259" = 6
  dimension "d260" = 1.5
  dimension "d261" = 1.5
  dimension "d262" = 1.5
  dimension "d263" = 1.5
  dimension "d264" = 6.4
  dimension "d265" = 4
  dimension "d266" = 10
  constraint horizontal L0
  constraint vertical L1
  constraint horizontal L2
  constraint vertical L3
  constraint horizontal L4
  constraint vertical L5
  constraint horizontal L6
  constraint vertical L7
  constraint coincident P1 L4
  constraint coincident P1 L5
  constraint coincident P0 L4
  constraint coincident P0 L7
  constraint horizontal L10
  constraint vertical L11
  constraint horizontal L12
  constraint vertical L13
  measures "d250" distance of L0.start L0.end
  measures "d251" distance of L0.start L2.end
  measures "d252" diameter of A0
  measures "d253" distance of L2 A0.centre
  measures "d254" distance of L1 A0.centre
  measures "d255" distance of P0 P1
  measures "d256" distance of P0 L6.end
  measures "d258" distance of L2 L6
  measures "d259" distance of L3 L7
  measures "d260" distance of P1 L4.end
  measures "d261" distance of P1 L5.start
  measures "d262" distance of P0 L4.start
  measures "d263" distance of P0 L7.end
  measures "d264" diameter of A1
  measures "d265" distance of L10.start L10.end
  measures "d266" distance of L10.start L12.end
extrude "Extrude32" add sketch "Sketch14" against normal blind 1.4 separate body contours L0 L1 L2 L3 | A0 | L4 L5 L6 L7 L8 L9 A1 | A1 | L5 L6 A1 | L10 L11 L12 L13 makes body 16
extrude "Extrude33" add sketch "Sketch14" along normal blind 1 separate body contours L4 L5 L6 L7 L8 L9 A1 | L5 L6 A1 makes body 17
extrude "Extrude34" add sketch "Sketch14" along normal blind 5.6 contours A1 bodies 16 17
fillet "Fillet6" radius 0.5 1 edges at (-18.6834, 132.9428, 5.6) on bodies 16
extrude "Extrude35" add sketch "Sketch14" along normal blind 1 contours L10 L11 L12 L13 bodies 16
extrude "Extrude36" cut sketch "Sketch14" against normal blind 2 contours A0 bodies 16
copy_body "Body->Comp6" bodies 16 removing the originals makes body 18 in component "MotorDriver2"
sketch "Sketch15" plane through (0, 0, 0) normal (0, 0, 1) x (1, 0, 0)
  line L0 (25, 125) -> (43.2, 125)
  line L1 (43.2, 125) -> (43.2, 94)
  line L2 (43.2, 94) -> (25, 94)
  line L3 (25, 94) -> (25, 125)
  line L4 (29.6, 126.4) -> (38.6, 126.4)
  line L5 (38.6, 126.4) -> (38.6, 119)
  line L6 (38.6, 119) -> (29.6, 119)
  line L7 (29.6, 119) -> (29.6, 126.4)
  circle A0 centre (27, 119) radius 1
  circle A1 centre (41, 119) radius 1
  line L8 (40, 115) -> (33, 115)
  line L9 (33, 115) -> (33, 108)
  line L10 (33, 108) -> (40, 108)
  line L11 (40, 108) -> (40, 115)
  dimension "d279" = 18.2
  dimension "d280" = 31
  dimension "d281" = 9
  dimension "d282" = 7.4
  dimension "d283" = 1.4
  dimension "d284" = 4.6
  dimension "d285" = 2
  dimension "d286" = 2
  dimension "d287" = 6
  dimension "d288" = 6
  constraint horizontal L0
  constraint vertical L1
  constraint horizontal L2
  constraint vertical L3
  constraint horizontal L4
  constraint vertical L5
  constraint horizontal L6
  constraint vertical L7
  constraint horizontal L8
  constraint vertical L9
  constraint horizontal L10
  constraint vertical L11
  measures "d279" distance of L0.start L0.end
  measures "d280" distance of L0.start L2.end
  measures "d281" distance of L4.start L4.end
  measures "d282" distance of L4.start L6.end
  measures "d283" distance of L0 L4
  measures "d284" distance of L1 L5
  measures "d285" diameter of A0
  measures "d286" diameter of A1
  measures "d287" distance of L0 A1.centre
  measures "d288" distance of L0 A0.centre
extrude "Extrude37" add sketch "Sketch15" against normal blind 1.4 separate body contours L0 L1 L2 L3 L5 L6 L7 | L0 L5 L6 L7 | L8 L9 L10 L11 makes body 19
extrude "Extrude38" add sketch "Sketch15" along normal blind 3 contours L8 L9 L10 L11 bodies 19
extrude "Extrude39" add sketch "Sketch15" along normal blind 3.4 separate body contours L0 L4 L5 L7 | L0 L5 L6 L7 makes body 20
fillet "Fillet7" radius 1.5 2 edges at (29.6, 122.7, 3.4) (38.6, 122.7, 3.4) on bodies 20
fillet "Fillet7" radius 1.5 2 edges at (29.6, 122.7, 0) (38.6, 122.7, 0) on bodies 20
combine "Combine2" operation add target body 19 tool bodies 20
copy_body "Body->Comp7" bodies 19 removing the originals makes body 21 in component "ChargeModule"
sketch "Sketch16" plane through (0, 0, 0) normal (0, 0, 1) x (1, 0, 0)
  line L0 (60, 80) -> (68.3, 80)
  line L1 (68.3, 80) -> (68.3, 67)
  line L2 (68.3, 67) -> (60, 67)
  line L3 (60, 67) -> (60, 80)
  line L4 (69.6, 65.7) -> (58.7, 65.7)
  line L5 (58.7, 65.7) -> (58.7, 81.3)
  line L6 (58.7, 81.3) -> (69.6, 81.3)
  line L7 (69.6, 81.3) -> (69.6, 65.7)
  line L8 (60.9, 67.9) -> (60.9, 79.1)
  line L9 (60.9, 79.1) -> (67.4, 79.1)
  line L10 (67.4, 79.1) -> (67.4, 67.9)
  line L11 (67.4, 67.9) -> (60.9, 67.9)
  line L12 (66.15, 79) -> (62.15, 79)
  line L13 (62.15, 79) -> (62.15, 78)
  line L14 (62.15, 78) -> (66.15, 78)
  line L15 (66.15, 78) -> (66.15, 79)
  line L16 (62.15, 73) -> (66.15, 73)
  line L17 (66.15, 74) -> (62.15, 74)
  line L18 (62.15, 74) -> (62.15, 73)
  line L19 (66.15, 73) -> (66.15, 74)
  dimension "d299" = 8.3
  dimension "d300" = 13
  dimension "d301" = -1.3
  dimension "d304" = 0.9
  dimension "d311" = 1
  dimension "d312" = 2.15
  constraint horizontal L0
  constraint vertical L1
  constraint horizontal L2
  constraint vertical L3
  constraint horizontal L12
  constraint vertical L13
  constraint horizontal L14
  constraint vertical L15
  constraint horizontal L17
  constraint vertical L18
  constraint horizontal L16
  constraint vertical L19
  measures "d299" distance of L0.start L0.end
  measures "d300" distance of L0.start L2.end
  measures "d311" distance of L0 L12
  measures "d312" distance of L1 L15
extrude "Extrude40" add sketch "Sketch16" against normal blind 9.5 separate body contours L0 L1 L2 L3 | L8 L9 L10 L11 | L12 L13 L14 L15 | L16 L17 L18 L19 makes body 22
extrude "Extrude41" add sketch "Sketch16" along normal blind 2 contours L0 L1 L2 L3 | L4 L5 L6 L7 bodies 22
chamfer "Chamfer2" distance 1.5 distance2 1.5 4 edges at (58.7, 73.5, 2) (64.15, 81.3, 2) (69.6, 73.5, 2) (64.15, 65.7, 2) measured on face at (59.4333, 75.3667, 2) measured on face at (59.4333, 75.3667, 2) measured on face at (59.4333, 75.3667, 2) measured on face at (59.4333, 75.3667, 2) on bodies 22
sketch "Sketch17" plane through (60.9, 0, 0) normal (1, 0, 0) x (0, 1, 0)
  line L0 (67.9, 0) -> (79.1, 0)
  line L1 (79.1, 0) -> (79.1, 2)
  line L2 (79.1, 2) -> (67.9, 2)
  line L3 (67.9, 2) -> (67.9, 0)
  line L4 (79.8, 2) -> (67.2, 2)
  line L5 (67.2, 2) -> (65.7, 0.5)
  line L6 (65.7, 0.5) -> (81.3, 0.5)
  line L7 (81.3, 0.5) -> (79.8, 2)
  line L8 (69.5, 2) -> (69.5, 4.7172)
  spline S0 degree 5 poles (67.9, 2) (67.9022, 2.0701) (67.9093, 2.209) (67.9277, 2.4132) (67.9681, 2.677) (68.0469, 2.9918) (68.1565, 3.2902) (68.2994, 3.571) (68.4768, 3.8335) (68.6875, 4.0784) (68.9287, 4.307) (69.1441, 4.478) (69.3175, 4.6) (69.4383, 4.6786) (69.5, 4.7172) knots 0 0 0 0 0 0 0.1 0.2 0.3 0.4 0.5 0.6 0.7 0.8 0.9 1 1 1 1 1 1
  spline S1 degree 5 poles (69.5, 4.7172) (69.6251, 4.6245) (69.8813, 4.4428) (70.284, 4.1807) (70.8581, 3.8524) (71.6418, 3.4799) (72.4966, 3.148) (73.4266, 2.8592) (74.4316, 2.6132) (75.506, 2.4069) (76.6436, 2.2367) (77.5996, 2.1268) (78.3406, 2.0581) (78.8451, 2.0184) (79.1, 2) knots 0 0 0 0 0 0 0.1 0.2 0.3 0.4 0.5 0.6 0.7 0.8 0.9 1 1 1 1 1 1
  point P0 (68.3042, 3.5599)
  point P1 (73, 3)
  constraint coincident L4 L8.start
  constraint perpendicular L4 L8
  constraint coincident L2.end L3.start
  constraint coincident L1.end L2.start
extrude "Extrude42" add sketch "Sketch17" along normal blind 6.5 separate body contours L2 L4 L8 S0 | L2 L4 L8 S1 makes body 23
combine "Combine3" operation add target body 22 tool bodies 23 keep tools
combine "Combine4" operation add target body 23 tool bodies 22
extrude "Extrude43" add sketch "Sketch16" against normal blind 15.7 separate body contours L12 L13 L14 L15 | L16 L17 L18 L19 makes body 24 at (64.8167, 78, -5.2333) makes body 25 at (63.4833, 74, -5.2333)
combine "Combine5" operation add target body 23 tool bodies 24 25
chamfer "Chamfer3" distance 0.5 distance2 0.5 2 edges at (62.15, 73.5, -15.7) (62.15, 78.5, -15.7) measured on face at (63.4833, 73.6667, -15.7) measured on face at (63.4833, 78.6667, -15.7) on bodies 23
chamfer "Chamfer3" distance 0.5 distance2 0.5 2 edges at (66.15, 73.5, -15.7) (66.15, 78.5, -15.7) measured on face at (63.4833, 73.6667, -15.7) measured on face at (63.4833, 78.6667, -15.7) on bodies 23
copy_body "Body->Comp8" bodies 23 removing the originals makes body 26 in component "PowerSwitcher"
sketch "Sketch18" plane through (0, 0, 0) normal (0, 1, 0) x (1, 0, 0)
  line L0 (85, -23) -> (105, -23)
  line L1 (105, -23) -> (105, -9)
  line L2 (105, -9) -> (85, -9)
  line L3 (85, -9) -> (85, -23)
  circle A0 centre (95, -16) radius 4
  circle A1 centre (95, -16) radius 5
  dimension "d319" = 14
  dimension "d320" = 8
  dimension "d321" = 7
  constraint horizontal L0
  constraint vertical L1
  constraint horizontal L2
  constraint vertical L3
  constraint concentric A0 A1
  measures "d319" distance of L0.start L2.end
  measures "d320" diameter of A0
  measures "d321" distance of L0 A0.centre